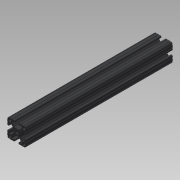
# Autodesk Inventor part: 1515-LITE
Saved by Autodesk Inventor 2013 (Build 170138000, 138)
## iProperties
Company: 80/20 Inc.
Created: 2014-04-23
Part Number: 1515-LITE
Material: Generic
Document SubType Name: Modeling
Density: 1 g/cm^3
Vendor: 80/20 Inc.
Engineer: Ross Bowman
Designer: Ross Bowman
Catalog Web Link: 8020.net
Material: 6105-T5 Aluminum
Author: Ross Bowman
Keywords: 80/20 , 8020 , T-Slot , Extrusion
Autodesk Inventor part; units mm, degrees
ref_plane "YZ Plane" through (0, 0, 0) normal (1, 0, 0) x (0, 1, 0)
ref_plane "XZ Plane" through (0, 0, 0) normal (0, 1, 0) x (-1, 0, 0)
ref_plane "XY Plane" through (0, 0, 0) normal (0, 0, 1) x (1, 0, 0)
sketch "Sketch1" plane through (0, 0, 0) normal (0, 0, 1) x (1, 0, 0)
  line L0 (16.891, -11.8618) -> (12.2428, -11.8618)
  arc A0 (17.272, -12.2428) -> (16.891, -11.8618) centre (16.891, -12.2428) ccw
  line L1 (17.272, -14.478) -> (17.272, -12.2428)
  arc A1 (14.478, -17.272) -> (17.272, -14.478) centre (14.478, -14.478) ccw
  line L2 (12.2428, -17.272) -> (14.478, -17.272)
  arc A2 (11.8618, -16.891) -> (12.2428, -17.272) centre (12.2428, -16.891) ccw
  line L3 (11.8618, -12.2428) -> (11.8618, -16.891)
  arc A3 (12.2428, -11.8618) -> (11.8618, -12.2428) centre (12.2428, -12.2428) ccw
  circle A4 centre (0, 0) radius 3.3274
  line L4 (14.478, 17.272) -> (12.2428, 17.272)
  arc A5 (17.272, 14.478) -> (14.478, 17.272) centre (14.478, 14.478) ccw
  line L5 (17.272, 12.2428) -> (17.272, 14.478)
  arc A6 (16.891, 11.8618) -> (17.272, 12.2428) centre (16.891, 12.2428) ccw
  line L6 (12.2428, 11.8618) -> (16.891, 11.8618)
  arc A7 (11.8618, 12.2428) -> (12.2428, 11.8618) centre (12.2428, 12.2428) ccw
  line L7 (11.8618, 16.891) -> (11.8618, 12.2428)
  arc A8 (12.2428, 17.272) -> (11.8618, 16.891) centre (12.2428, 16.891) ccw
  line L8 (-14.478, -17.272) -> (-12.2428, -17.272)
  arc A9 (-17.272, -14.478) -> (-14.478, -17.272) centre (-14.478, -14.478) ccw
  line L9 (-17.272, -12.2428) -> (-17.272, -14.478)
  arc A10 (-16.891, -11.8618) -> (-17.272, -12.2428) centre (-16.891, -12.2428) ccw
  line L10 (-12.2428, -11.8618) -> (-16.891, -11.8618)
  arc A11 (-11.8618, -12.2428) -> (-12.2428, -11.8618) centre (-12.2428, -12.2428) ccw
  line L11 (-11.8618, -16.891) -> (-11.8618, -12.2428)
  arc A12 (-12.2428, -17.272) -> (-11.8618, -16.891) centre (-12.2428, -16.891) ccw
  line L12 (-16.891, 11.8618) -> (-12.2428, 11.8618)
  arc A13 (-17.272, 12.2428) -> (-16.891, 11.8618) centre (-16.891, 12.2428) ccw
  line L13 (-17.272, 14.478) -> (-17.272, 12.2428)
  arc A14 (-14.478, 17.272) -> (-17.272, 14.478) centre (-14.478, 14.478) ccw
  line L14 (-12.2428, 17.272) -> (-14.478, 17.272)
  arc A15 (-11.8618, 16.891) -> (-12.2428, 17.272) centre (-12.2428, 16.891) ccw
  line L15 (-11.8618, 12.2428) -> (-11.8618, 16.891)
  arc A16 (-12.2428, 11.8618) -> (-11.8618, 12.2428) centre (-12.2428, 12.2428) ccw
  arc A17 (-10.287, 12.7802) -> (-10.0267, 12.1519) centre (-9.3985, 12.7802) ccw
  line L16 (-10.287, 12.7802) -> (-10.287, 14.5547)
  arc A18 (-9.017, 15.8247) -> (-10.287, 14.5547) centre (-9.017, 14.5547) ccw
  line L17 (-9.017, 15.8247) -> (-6.8141, 15.8247)
  line L18 (-6.8141, 15.8247) -> (-6.8141, 14.986)
  line L19 (-6.8141, 14.986) -> (-5.6388, 14.986)
  arc A19 (-5.6388, 14.986) -> (-4.064, 16.5608) centre (-5.6388, 16.5608) ccw
  line L20 (-4.064, 16.5608) -> (-4.064, 17.4752)
  arc A20 (-4.064, 17.4752) -> (-5.6388, 19.05) centre (-5.6388, 17.4752) ccw
  line L21 (-5.6388, 19.05) -> (-7.9756, 19.05)
  arc A21 (-9.4996, 19.05) -> (-7.9756, 19.05) centre (-8.7376, 19.05) ccw
  line L22 (-9.4996, 19.05) -> (-14.3256, 19.05)
  arc A22 (-15.8496, 19.05) -> (-14.3256, 19.05) centre (-15.0876, 19.05) ccw
  line L23 (-15.8496, 19.05) -> (-15.875, 19.05)
  arc A23 (-15.875, 19.05) -> (-19.05, 15.875) centre (-15.875, 15.875) ccw
  line L24 (-19.05, 15.875) -> (-19.05, 15.8496)
  arc A24 (-19.05, 14.3256) -> (-19.05, 15.8496) centre (-19.05, 15.0876) ccw
  line L25 (-19.05, 14.3256) -> (-19.05, 9.4996)
  arc A25 (-19.05, 7.9756) -> (-19.05, 9.4996) centre (-19.05, 8.7376) ccw
  line L26 (-19.05, 7.9756) -> (-19.05, 5.6388)
  arc A26 (-19.05, 5.6388) -> (-17.4752, 4.064) centre (-17.4752, 5.6388) ccw
  line L27 (-17.4752, 4.064) -> (-16.5608, 4.064)
  arc A27 (-16.5608, 4.064) -> (-14.986, 5.6388) centre (-16.5608, 5.6388) ccw
  line L28 (-14.986, 5.6388) -> (-14.986, 6.7506)
  line L29 (-14.986, 6.7506) -> (-15.879, 6.7506)
  line L30 (-15.879, 6.7506) -> (-15.879, 8.9192)
  arc A28 (-14.609, 10.1892) -> (-15.879, 8.9192) centre (-14.609, 8.9192) ccw
  line L31 (-14.609, 10.1892) -> (-12.7428, 10.1892)
  arc A29 (-12.1142, 9.9289) -> (-12.7428, 10.1892) centre (-12.7428, 9.3002) ccw
  line L32 (-12.1142, 9.9289) -> (-8.1479, 5.9632)
  arc A30 (-6.7564, 2.6043) -> (-8.1479, 5.9632) centre (-11.5062, 2.6043) ccw
  line L33 (-6.7564, 2.6043) -> (-6.7564, -2.6043)
  arc A31 (-8.1479, -5.9632) -> (-6.7564, -2.6043) centre (-11.5062, -2.6043) ccw
  line L34 (-8.1479, -5.9632) -> (-12.1142, -9.9289)
  arc A32 (-12.7428, -10.1892) -> (-12.1142, -9.9289) centre (-12.7428, -9.3002) ccw
  line L35 (-12.7428, -10.1892) -> (-14.609, -10.1892)
  arc A33 (-15.879, -8.9192) -> (-14.609, -10.1892) centre (-14.609, -8.9192) ccw
  line L36 (-15.879, -8.9192) -> (-15.879, -6.7506)
  line L37 (-15.879, -6.7506) -> (-14.986, -6.7506)
  line L38 (-14.986, -6.7506) -> (-14.986, -5.6388)
  arc A34 (-14.986, -5.6388) -> (-16.5608, -4.064) centre (-16.5608, -5.6388) ccw
  line L39 (-16.5608, -4.064) -> (-17.4752, -4.064)
  arc A35 (-17.4752, -4.064) -> (-19.05, -5.6388) centre (-17.4752, -5.6388) ccw
  line L40 (-19.05, -5.6388) -> (-19.05, -7.9756)
  arc A36 (-19.05, -9.4996) -> (-19.05, -7.9756) centre (-19.05, -8.7376) ccw
  line L41 (-19.05, -9.4996) -> (-19.05, -14.3256)
  arc A37 (-19.05, -15.8496) -> (-19.05, -14.3256) centre (-19.05, -15.0876) ccw
  line L42 (-19.05, -15.8496) -> (-19.05, -15.875)
  arc A38 (-19.05, -15.875) -> (-15.875, -19.05) centre (-15.875, -15.875) ccw
  line L43 (-15.875, -19.05) -> (-15.8496, -19.05)
  arc A39 (-14.3256, -19.05) -> (-15.8496, -19.05) centre (-15.0876, -19.05) ccw
  line L44 (-14.3256, -19.05) -> (-9.4996, -19.05)
  arc A40 (-7.9756, -19.05) -> (-9.4996, -19.05) centre (-8.7376, -19.05) ccw
  line L45 (-7.9756, -19.05) -> (-5.6388, -19.05)
  arc A41 (-5.6388, -19.05) -> (-4.064, -17.4752) centre (-5.6388, -17.4752) ccw
  line L46 (-4.064, -17.4752) -> (-4.064, -16.5608)
  arc A42 (-4.064, -16.5608) -> (-5.6388, -14.986) centre (-5.6388, -16.5608) ccw
  line L47 (-5.6388, -14.986) -> (-6.8141, -14.986)
  line L48 (-6.8141, -14.986) -> (-6.8141, -15.8247)
  line L49 (-6.8141, -15.8247) -> (-9.017, -15.8247)
  arc A43 (-10.287, -14.5547) -> (-9.017, -15.8247) centre (-9.017, -14.5547) ccw
  line L50 (-10.287, -14.5547) -> (-10.287, -12.7802)
  arc A44 (-10.0267, -12.1519) -> (-10.287, -12.7802) centre (-9.3985, -12.7802) ccw
  line L51 (-10.0267, -12.1519) -> (-6.0215, -8.1473)
  arc A45 (-2.6631, -6.7564) -> (-6.0215, -8.1473) centre (-2.6631, -11.5062) ccw
  line L52 (-2.6631, -6.7564) -> (2.6631, -6.7564)
  arc A46 (6.0215, -8.1473) -> (2.6631, -6.7564) centre (2.6631, -11.5062) ccw
  line L53 (6.0215, -8.1473) -> (10.0267, -12.1519)
  arc A47 (10.287, -12.7802) -> (10.0267, -12.1519) centre (9.3985, -12.7802) ccw
  line L54 (10.287, -12.7802) -> (10.287, -14.5547)
  arc A48 (9.017, -15.8247) -> (10.287, -14.5547) centre (9.017, -14.5547) ccw
  line L55 (9.017, -15.8247) -> (6.8141, -15.8247)
  line L56 (6.8141, -15.8247) -> (6.8141, -14.986)
  line L57 (6.8141, -14.986) -> (5.6388, -14.986)
  arc A49 (5.6388, -14.986) -> (4.064, -16.5608) centre (5.6388, -16.5608) ccw
  line L58 (4.064, -16.5608) -> (4.064, -17.4752)
  arc A50 (4.064, -17.4752) -> (5.6388, -19.05) centre (5.6388, -17.4752) ccw
  line L59 (5.6388, -19.05) -> (7.9756, -19.05)
  arc A51 (9.4996, -19.05) -> (7.9756, -19.05) centre (8.7376, -19.05) ccw
  line L60 (9.4996, -19.05) -> (14.3256, -19.05)
  arc A52 (15.8496, -19.05) -> (14.3256, -19.05) centre (15.0876, -19.05) ccw
  line L61 (15.8496, -19.05) -> (15.875, -19.05)
  arc A53 (15.875, -19.05) -> (19.05, -15.875) centre (15.875, -15.875) ccw
  line L62 (19.05, -15.875) -> (19.05, -15.8496)
  arc A54 (19.05, -14.3256) -> (19.05, -15.8496) centre (19.05, -15.0876) ccw
  line L63 (19.05, -14.3256) -> (19.05, -9.4996)
  arc A55 (19.05, -7.9756) -> (19.05, -9.4996) centre (19.05, -8.7376) ccw
  line L64 (19.05, -7.9756) -> (19.05, -5.6388)
  arc A56 (19.05, -5.6388) -> (17.4752, -4.064) centre (17.4752, -5.6388) ccw
  line L65 (17.4752, -4.064) -> (16.5608, -4.064)
  arc A57 (16.5608, -4.064) -> (14.986, -5.6388) centre (16.5608, -5.6388) ccw
  line L66 (14.986, -5.6388) -> (14.986, -6.7506)
  line L67 (14.986, -6.7506) -> (15.879, -6.7506)
  line L68 (15.879, -6.7506) -> (15.879, -8.9192)
  arc A58 (14.609, -10.1892) -> (15.879, -8.9192) centre (14.609, -8.9192) ccw
  line L69 (14.609, -10.1892) -> (12.7428, -10.1892)
  arc A59 (12.1142, -9.9289) -> (12.7428, -10.1892) centre (12.7428, -9.3002) ccw
  line L70 (12.1142, -9.9289) -> (8.1479, -5.9632)
  arc A60 (6.7564, -2.6043) -> (8.1479, -5.9632) centre (11.5062, -2.6043) ccw
  line L71 (6.7564, -2.6043) -> (6.7564, 2.6043)
  arc A61 (8.1479, 5.9632) -> (6.7564, 2.6043) centre (11.5062, 2.6043) ccw
  line L72 (8.1479, 5.9632) -> (12.1142, 9.9289)
  arc A62 (12.7428, 10.1892) -> (12.1142, 9.9289) centre (12.7428, 9.3002) ccw
  line L73 (12.7428, 10.1892) -> (14.609, 10.1892)
  arc A63 (15.879, 8.9192) -> (14.609, 10.1892) centre (14.609, 8.9192) ccw
  line L74 (15.879, 8.9192) -> (15.879, 6.7506)
  line L75 (15.879, 6.7506) -> (14.986, 6.7506)
  line L76 (14.986, 6.7506) -> (14.986, 5.6388)
  arc A64 (14.986, 5.6388) -> (16.5608, 4.064) centre (16.5608, 5.6388) ccw
  line L77 (16.5608, 4.064) -> (17.4752, 4.064)
  arc A65 (17.4752, 4.064) -> (19.05, 5.6388) centre (17.4752, 5.6388) ccw
  line L78 (19.05, 5.6388) -> (19.05, 7.9756)
  arc A66 (19.05, 9.4996) -> (19.05, 7.9756) centre (19.05, 8.7376) ccw
  line L79 (19.05, 9.4996) -> (19.05, 14.3256)
  arc A67 (19.05, 15.8496) -> (19.05, 14.3256) centre (19.05, 15.0876) ccw
  line L80 (19.05, 15.8496) -> (19.05, 15.875)
  arc A68 (19.05, 15.875) -> (15.875, 19.05) centre (15.875, 15.875) ccw
  line L81 (15.875, 19.05) -> (15.8496, 19.05)
  arc A69 (14.3256, 19.05) -> (15.8496, 19.05) centre (15.0876, 19.05) ccw
  line L82 (14.3256, 19.05) -> (9.4996, 19.05)
  arc A70 (7.9756, 19.05) -> (9.4996, 19.05) centre (8.7376, 19.05) ccw
  line L83 (7.9756, 19.05) -> (5.6388, 19.05)
  arc A71 (5.6388, 19.05) -> (4.064, 17.4752) centre (5.6388, 17.4752) ccw
  line L84 (4.064, 17.4752) -> (4.064, 16.5608)
  arc A72 (4.064, 16.5608) -> (5.6388, 14.986) centre (5.6388, 16.5608) ccw
  line L85 (5.6388, 14.986) -> (6.8141, 14.986)
  line L86 (6.8141, 14.986) -> (6.8141, 15.8247)
  line L87 (6.8141, 15.8247) -> (9.017, 15.8247)
  arc A73 (10.287, 14.5547) -> (9.017, 15.8247) centre (9.017, 14.5547) ccw
  line L88 (10.287, 14.5547) -> (10.287, 12.7802)
  arc A74 (10.0267, 12.1519) -> (10.287, 12.7802) centre (9.3985, 12.7802) ccw
  line L89 (10.0267, 12.1519) -> (6.0215, 8.1473)
  arc A75 (2.6631, 6.7564) -> (6.0215, 8.1473) centre (2.6631, 11.5062) ccw
  line L90 (2.6631, 6.7564) -> (-2.6631, 6.7564)
  arc A76 (-6.0215, 8.1473) -> (-2.6631, 6.7564) centre (-2.6631, 11.5062) ccw
  line L91 (-6.0215, 8.1473) -> (-10.0267, 12.1519)
  constraints: 184 end point, 152 point on circle, 77 centre point
extrude "Extrusion1" add sketch "Sketch1" against normal blind 304.8
body "Solid1"
